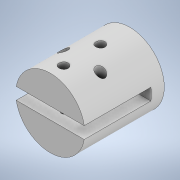
# Autodesk Inventor part: Claw_Attachment
Saved by Autodesk Inventor 2022 (Build 260153000, 153)
## iProperties
Created: 2022-02-27
Part Number: Claw_Attachment
Material: Generic
Document SubType Name: Modeling
Designer: Mlees
Density: 1 g/cm^3
Appearance: Default
Author: Mlees
Autodesk Inventor part; units mm, degrees
ref_plane "YZ Plane" through (0, 0, 0) normal (1, 0, 0) x (0, 1, 0)
sketch "Sketch1" plane through (0, 0, 0) normal (0, 0, 1) x (1, 0, 0)
  circle A0 centre (0, 0) radius 18.75
  constraints: 1 centre point, 1 coincident
extrude "Extrusion1" add sketch "Sketch1" along normal blind 7
sketch "Sketch2" plane through (0, 0, 7) normal (0, 0, 1) x (1, 0, 0)
  line L0 (0, -3.25) -> (-18.4662, -3.25)
  circle A0 centre (0, 0) radius 18.75 projected
  line L1 (0, 3.25) -> (-18.4662, 3.25)
  line L2 (0, 3.25) -> (18.4662, 3.25)
  line L3 (0, -3.25) -> (18.4662, -3.25)
  arc A1 (18.4662, 3.25) -> (-18.4662, 3.25) centre (0, 0) ccw
  arc A2 (-18.4662, -3.25) -> (18.4662, -3.25) centre (0, 0) ccw
  dimension "d3" = 3.25
  dimension "d4" = 3.25
  constraints: 8 end point, 8 point on circle, 2 centre point, 2 concentric, 2 point on line, 1 horizontal, 1 parallel
  measures "d3" distance of point (0, 0) L1.start
  measures "d4" distance of point (0, 0) L0.start
extrude "Extrusion2" add sketch "Sketch2" along normal blind 31.2 contours L3 A0 L0 | A0 L2 L1
ref_plane "Work Plane1" through (0, 18.75, 0) normal (0, -1, 0) x (1, 0, 0)
sketch "Sketch3" plane through (0, 18.75, 0) normal (0, -1, 0) x (1, 0, 0)
  line L0 (-18.4662, 7) -> (18.4662, 7) projected
  circle A0 centre (0, 16) radius 1.25
  circle A1 centre (0, 36) radius 1.25
  circle A2 centre (10, 26) radius 1.25
  circle A3 centre (-10, 26) radius 1.25
  circle A4 centre (0, 36) radius 1.25
  circle A5 centre (0, 16) radius 1.25
  circle A6 centre (-10, 26) radius 1.25
  circle A7 centre (10, 26) radius 1.25
  point P0 (0, 0)
  point P1 (0, 26)
  dimension "d8" = 2.5
  dimension "d12" = 360
  constraints: 8 centre point, 17 other
  measures "d8" diameter of A0
ref_plane "Work Plane2" through (0, -18.75, 0) normal (0, 1, 0) x (1, 0, 0)
extrude "Extrusion3" cut sketch "Sketch3" along normal up to surface (37.5 mm away)
sketch "Sketch4" plane through (0, 18.75, 0) normal (0, -1, 0) x (1, 0, 0)
  circle A0 centre (0, 16) radius 1.25 projected
  circle A1 centre (0, 16) radius 2.5
  circle A2 centre (10, 26) radius 1.25 projected
  circle A3 centre (10, 26) radius 2.5
  circle A4 centre (0, 36) radius 1.25 projected
  circle A5 centre (0, 36) radius 2.5
  circle A6 centre (-10, 26) radius 1.25 projected
  circle A7 centre (-10, 26) radius 2.5
  point P0 (0, 0)
  dimension "d16" = 5
  dimension "d17" = 5
  constraints: 4 centre point, 4 coincident
  measures "d16" diameter of A1
  measures "d17" diameter of A3
sketch "Sketch5" plane through (0, 0, 38.2) normal (0, 0, 1) x (1, 0, 0)
  arc A0 (18.4662, -3.25) -> (18.4662, 3.25) centre (0, 0) ccw projected
  arc A1 (-18.4662, 3.25) -> (-18.4662, -3.25) centre (0, 0) ccw projected
  arc A2 (18.4662, 3.25) -> (-18.4662, 3.25) centre (0, 0) ccw
  line L0 (-18.4662, -3.25) -> (18.4662, -3.25)
  line L1 (18.4662, 3.25) -> (-18.4662, 3.25) projected
  line L2 (18.4662, 3.25) -> (-18.4662, 3.25)
  line L3 (18.4662, -3.25) -> (-18.4662, -3.25) projected
  arc A3 (-18.4662, -3.25) -> (18.4662, -3.25) centre (0, 0) ccw
  constraints: 4 end point, 4 point on circle, 2 centre point, 1 collinear, 1 concentric, 1 horizontal
extrude "Extrusion4" add sketch "Sketch5" along normal blind 5 contours A3 L0 | L1 A2
extrude "Extrusion5" cut sketch "Sketch4" along normal blind 8
sketch "Sketch6" plane through (0, 0, 0) normal (0, 0, -1) x (-1, 0, 0)
  arc A0 (0, -2.75) -> (0, 2.75) centre (0, 0) ccw
  line L0 (0, -2.75) -> (0, 2.75)
  dimension "d22" = 5.5
  constraints: 2 end point, 2 point on circle, 1 centre point, 1 coincident, 1 vertical
  measures "d22" diameter of A0
extrude "Extrusion6" cut sketch "Sketch6" against normal blind 6.2
body "Solid1"
